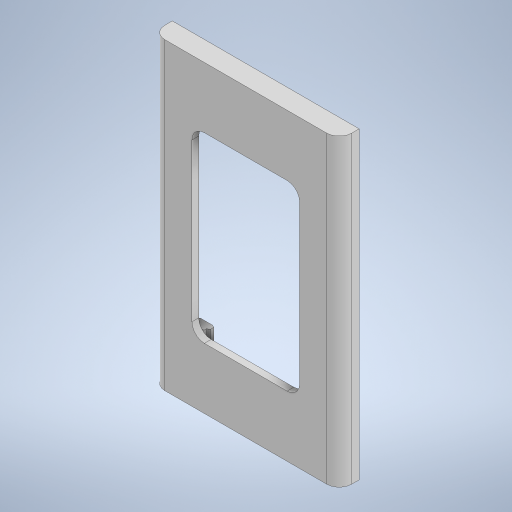
# Autodesk Inventor part: 스위치 커버
Saved by Autodesk Inventor 2023 (Build 270158000, 158)
## iProperties
Created: 2022-06-24
Part Number: 스위치 커버
Material: 일반
Document SubType Name: Modeling
Designer: user
Density: 1 g/cm^3
Appearance: 기본값
Author: user
Autodesk Inventor part; units mm, degrees
ref_plane "YZ Plane" through (0, 0, 0) normal (1, 0, 0) x (0, 1, 0)
ref_plane "XZ Plane" through (0, 0, 0) normal (0, 1, 0) x (-1, 0, 0)
ref_plane "XY Plane" through (0, 0, 0) normal (0, 0, 1) x (1, 0, 0)
sketch "스케치1" plane through (0, 0, 0) normal (0, 0, 1) x (1, 0, 0)
  line L0 (-37.5, 61) -> (37.5, 61)
  line L1 (37.5, 61) -> (37.5, -61)
  line L2 (37.5, -61) -> (-37.5, -61)
  line L3 (-37.5, -61) -> (-37.5, 61)
  line L4 (-37.5, 61) -> (37.5, -61) construction
  line L5 (37.5, 61) -> (-37.5, -61) construction
  line L6 (-21.6, 36.6) -> (21.6, 36.6)
  line L7 (21.6, 36.6) -> (21.6, -36.6)
  line L8 (21.6, -36.6) -> (-21.6, -36.6)
  line L9 (-21.6, -36.6) -> (-21.6, 36.6)
  line L10 (-21.6, 36.6) -> (21.6, -36.6) construction
  line L11 (21.6, 36.6) -> (-21.6, -36.6) construction
  point P0 (0, 0)
  dimension "d0" = 75
  dimension "d1" = 122
  dimension "d2" = 43.2
  dimension "d3" = 73.2
  constraints: 24 end point, 4 midpoint, 4 parallel, 2 horizontal, 2 perpendicular
  measures "d0" distance of L1.end L2.end
  measures "d1" distance of L0.end L1.end
  measures "d2" distance of L7.end L8.end
  measures "d3" distance of L6.end L7.end
extrude "돌출1" add sketch "스케치1" along normal blind 8
fillet "모깎기1" radius 5 2 edges at (37.5, 0, 8) (-37.5, 0, 8)
shell "쉘1" thickness 1.7 removed faces 1 at (32.2, -12.2, 0)
sketch "스케치2" plane through (32.5, 59.3, 6.3) normal (0, 0, -1) x (-1, 0, 0)
  line L0 (6.4857, -104.5153) -> (58.5143, -104.5153)
  line L1 (58.5143, -104.5153) -> (58.5143, -14.0847)
  line L2 (58.5143, -14.0847) -> (6.4857, -14.0847)
  line L3 (6.4857, -14.0847) -> (6.4857, -104.5153)
  line L4 (6.4857, -104.5153) -> (58.5143, -14.0847) construction
  line L5 (58.5143, -104.5153) -> (6.4857, -14.0847) construction
  point P0 (32.5, -59.3)
  constraints: 12 end point, 2 midpoint, 2 parallel, 1 horizontal, 1 perpendicular
extrude "돌출2" cut sketch "스케치2" along normal blind 8
sketch "스케치3" plane through (32.5, 59.3, 6.3) normal (0, 0, -1) x (-1, 0, 0)
  line L0 (54, -15.55) -> (61, -15.55)
  line L1 (61, -15.55) -> (61, -22.45)
  line L2 (61, -22.45) -> (54, -22.45)
  line L3 (54, -22.45) -> (54, -15.55)
  line L4 (54, -15.55) -> (61, -22.45) construction
  line L5 (61, -15.55) -> (54, -22.45) construction
  line L6 (54, -15.55) -> (57.5, -15.55)
  line L7 (57.5, -15.55) -> (57.5, -22.45)
  line L8 (57.5, -22.45) -> (54, -22.45)
  line L9 (54, -22.45) -> (54, -15.55)
  point P0 (32.5, -59.3)
  point P1 (57.5, -19)
  dimension "d10" = 36.85
  dimension "d11" = 6.9
  dimension "d12" = 7
  dimension "d13" = 21.5
  constraints: 20 end point, 4 parallel, 3 midpoint, 2 horizontal, 2 perpendicular
  measures "d10" distance from line of point (32.5, -59.3) L2
  measures "d11" distance of L0.end L1.end
  measures "d12" distance of L0.start L0.end
  measures "d13" distance from line of point (32.5, -59.3) L3
extrude "돌출3" add sketch "스케치3" along normal blind 6.5 contours L0 L7 L2 L3
chamfer "모따기1" distance 2 angle 45 1 edges at (-25, 40.3, -0.2)
sketch "스케치4" plane through (-25, 36.85, 6.3) normal (0, -1, 0) x (1, 0, 0)
  line L0 (2, -6.5) -> (3.5, -6.5) projected
  line L1 (4.5, -4.5774) -> (3.5, -4)
  line L2 (3.5, 0) -> (3.5, -6.5) projected
  line L3 (4.5, -4.5774) -> (4.5, -5.9226)
  line L4 (4.5, -5.9226) -> (3.5, -6.5)
  line L5 (0, -4.5) -> (2, -6.5) projected
  line L6 (0, -4.5) -> (-4.5, 0)
  line L7 (-4.5, 0) -> (0, 0)
  line L8 (0, 0) -> (3.5, 0)
  line L9 (57.5, 0) -> (-7.5, 0) projected
  line L10 (2, -6.5) -> (-4.5, -6.5)
  line L11 (-4.5, 0) -> (-4.5, -6.5)
  point P0 (25, -6.3)
  dimension "d19" = 4
  dimension "d23" = 1
  dimension "d24" = 60
  dimension "d25" = 60
  constraints: 17 end point, 2 collinear, 2 horizontal, 1 perpendicular, 1 point on line, 1 vertical
  measures "d19" distance of L2.start L1.end
  measures "d23" distance between parallel lines of L2 L3
  measures "d24" angle of L2 L1
  measures "d25" angle of L2 L4
extrude "돌출4" add sketch "스케치4" against normal blind 7.3
mirror "미러1" about plane through (0, 0, 0) normal (0, 1, 0) of "돌출4", "돌출3", "모따기1"
mirror "미러2" about plane through (0, 0, 0) normal (1, 0, 0) of "돌출4", "돌출3", "모따기1", "미러1"
sketch "스케치5" plane through (32.5, 59.3, 6.3) normal (0, 0, -1) x (-1, 0, 0)
  line L0 (57.5, -104.3) -> (7.5, -104.3)
  line L1 (7.5, -104.3) -> (7.5, -14.3)
  line L2 (7.5, -14.3) -> (57.5, -14.3)
  line L3 (57.5, -14.3) -> (57.5, -104.3)
  line L4 (57.5, -104.3) -> (7.5, -14.3) construction
  line L5 (7.5, -104.3) -> (57.5, -14.3) construction
  point P0 (32.5, -59.3)
  dimension "d28" = 50
  dimension "d29" = 90
  constraints: 12 end point, 2 midpoint, 2 parallel, 1 horizontal, 1 perpendicular
  measures "d28" distance of L1.end L2.end
  measures "d29" distance of L0.end L1.end
fillet "모깎기6" radius 5 4 edges at (-21.6, 36.6, 7.15) (21.6, 36.6, 7.15) (21.6, -36.6, 7.15) (-21.6, -36.6, 7.15)
chamfer "모따기2" distance 3 angle 45 4 edges at (29.5, 40.5, -0.2) (-29.5, 40.5, -0.2) (29.5, -40.5, -0.2) (-29.5, -40.5, -0.2)
thicken "두껍게 하기1" operation add thickness 1 both sides no extend neighbours no toward (0, 0, -1) faces at (7.1667, -54.25, 6.3)
fillet "모깎기7" radius 2 12 edges at (25.5, -44.15, 5.3) (-25.5, -44.15, 5.3) (-25.5, 36.85, 5.3) (25.5, 36.85, 5.3) (29.5, 40.5, 5.3) (29.5, -40.5, 5.3) (-29.5, -40.5, 5.3) (-29.5, 40.5, 5.3) (25.5, -36.85, 5.3) (-25.5, -36.85, 5.3) (-25.5, 44.15, 5.3) (25.5, 44.15, 5.3)
